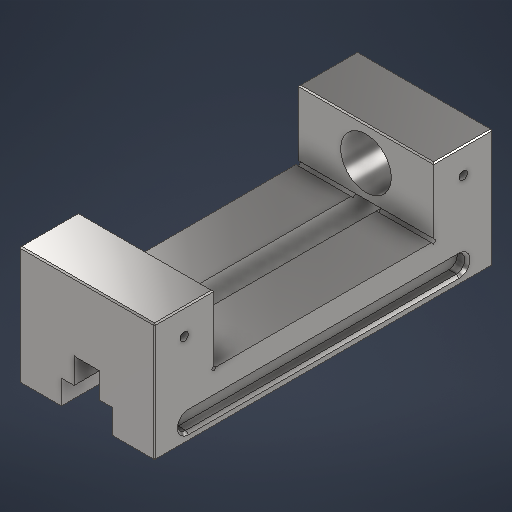
# Autodesk Inventor part: Part1
Saved by Autodesk Inventor 2026 (Build 300175000, 175)
## iProperties
Created: 2026-03-22
Part Number: Part1
Material: Generic
Document SubType Name: Modeling
Designer: Mlinč
Density: 1 g/cm^3
Appearance: Default
Author: Mlinč
Autodesk Inventor part; units mm, degrees
ref_plane "XZ Plane" through (0, 0, 0) normal (0, 1, 0) x (-1, 0, 0)
ref_plane "XY Plane" through (0, 0, 0) normal (0, 0, 1) x (1, 0, 0)
sketch "Sketch1" plane through (0, 0, 0) normal (0, 1, 0) x (-1, 0, 0)
  line L0 (0, 0) -> (80, 0)
  line L1 (80, 0) -> (80, -200)
  line L2 (80, -200) -> (0, -200)
  line L3 (0, -200) -> (0, 0)
  dimension "d0" = 80
  dimension "d1" = 200
  constraints: 8 end point, 2 parallel, 1 horizontal, 1 perpendicular
  measures "d0" distance of L0.start L0.end
  measures "d1" distance of L0.end L1.end
extrude "Extrusion1" add sketch "Sketch1" along normal blind 70
sketch "Sketch2" plane through (0, 0, 0) normal (1, 0, 0) x (0, 0, -1)
  line L0 (200, 70) -> (0, 70) projected
  line L1 (35, 70) -> (165, 70)
  line L2 (165, 70) -> (165, 30)
  line L3 (165, 30) -> (35, 30)
  line L4 (35, 30) -> (35, 70)
  line L5 (0, 0) -> (0, 70) projected
  line L6 (200, 0) -> (200, 70) projected
  dimension "d4" = 35
  dimension "d5" = 35
  dimension "d6" = 40
  constraints: 8 end point, 2 parallel, 1 horizontal, 1 perpendicular, 1 point on line
  measures "d4" distance between parallel lines of L5 L4
  measures "d5" distance between parallel lines of L6 L2
  measures "d6" distance of L3.end L1.start
extrude "Extrusion2" cut sketch "Sketch2" against normal through all
sketch "Sketch3" plane through (0, 0, -200) normal (0, 0, -1) x (-1, 0, 0)
  line L0 (80, 0) -> (0, 0) projected
  line L1 (25, 0) -> (25, 15)
  line L2 (25, 15) -> (32.5, 15)
  line L3 (32.5, 15) -> (32.5, 30)
  line L4 (32.5, 30) -> (47.5, 30)
  line L5 (47.5, 30) -> (47.5, 15)
  line L6 (47.5, 15) -> (55, 15)
  line L7 (55, 15) -> (55, 0)
  line L8 (40, 0) -> (40, 70) construction
  line L9 (80, 70) -> (0, 70) projected
  dimension "d9" = 15
  dimension "d10" = 15
  dimension "d11" = 30
  dimension "d12" = 15
  constraints: 16 end point, 5 perpendicular, 4 point on line, 2 midpoint, 1 collinear, 1 vertical, 1 other
  measures "d9" distance of L3.end L4.end
  measures "d10" distance of L1.start L1.end
  measures "d11" distance between parallel lines of L7 L1
  measures "d12" distance of L4.end L5.end
extrude "Extrusion3" cut sketch "Sketch3" against normal through all
sketch "Sketch4" plane through (0, 70, -200) normal (0, 0, -1) x (-1, 0, 0)
  circle A0 centre (40, -20) radius 15
  line L0 (0, 0) -> (80, 0) projected
  point P0 (0, -70)
  point P1 (40, 0)
  dimension "d15" = 20
  dimension "d16" = 30
  constraints: 1 centre point, 1 midpoint, 1 vertical alignment
  measures "d15" distance from line of L0 A0.centre
  measures "d16" diameter of A0
extrude "Extrusion4" cut sketch "Sketch4" against normal up to surface (35 mm away)
sketch "Sketch5" plane through (0, 0, 0) normal (1, 0, 0) x (0, 0, -1)
  line L0 (20, 10) -> (180, 10) construction
  line L1 (200, 15) -> (0, 15) projected
  line L2 (20, 5) -> (180, 5)
  line L3 (180, 15) -> (20, 15)
  arc A0 (20, 15) -> (20, 5) centre (20, 10) ccw
  arc A1 (180, 5) -> (180, 15) centre (180, 10) ccw
  line L4 (0, 0) -> (200, 0) projected
  line L5 (0, 0) -> (0, 70) projected
  point P0 (100, 10)
  dimension "d19" = 5
  dimension "d20" = 160
  dimension "d21" = 5
  dimension "d22" = 20
  constraints: 8 end point, 4 point on circle, 4 tangent, 2 centre point, 2 parallel, 1 midpoint
  measures "d19" radius of A0
  measures "d20" distance of L3.start L3.end
  measures "d21" distance between parallel lines of L2 L4
  measures "d22" distance from line of L5 L0.start
extrude "Extrusion5" cut sketch "Sketch5" against normal blind 6
ref_plane "Work Plane1" through (-40, 0, 0) normal (1, 0, 0) x (0, 1, 0)
mirror "Mirror1" about plane through (-40, 0, 0) normal (1, 0, 0) of "Extrusion5"
sketch "Sketch6" plane through (0, 0, 0) normal (1, 0, 0) x (0, 0, -1)
  line L0 (35, 28.5858) -> (33.5858, 30)
  line L1 (33.5858, 30) -> (35, 31.4142)
  line L2 (35, 31.4142) -> (36.4142, 30)
  line L3 (36.4142, 30) -> (35, 28.5858)
  line L4 (165, 30) -> (35, 30) projected
  line L5 (35, 28.5858) -> (35, 31.4142) construction
  line L6 (33.5858, 30) -> (36.4142, 30) construction
  line L7 (165, 28.5858) -> (166.4142, 30)
  line L8 (166.4142, 30) -> (165, 31.4142)
  line L9 (165, 31.4142) -> (163.5858, 30)
  line L10 (163.5858, 30) -> (165, 28.5858)
  line L11 (165, 28.5858) -> (165, 31.4142) construction
  line L12 (166.4142, 30) -> (163.5858, 30) construction
  point P0 (0, 0)
  dimension "d26" = 2
  constraints: 24 end point, 5 perpendicular, 4 midpoint, 4 parallel, 2 horizontal
  measures "d26" distance of L1.end L2.end
extrude "Extrusion6" cut sketch "Sketch6" against normal through all
sketch "Sketch7" plane through (0, 0, 0) normal (1, 0, 0) x (0, 0, -1)
  circle A0 centre (17.5, 55) radius 2.5
  circle A1 centre (182.5, 55) radius 2.5
  line L0 (0, 70) -> (35, 70) projected
  line L1 (0, 0) -> (0, 70) projected
  line L2 (200, 0) -> (200, 70) projected
  dimension "d30" = 5
  dimension "d31" = 15
  dimension "d32" = 17.5
  dimension "d33" = 17.5
  constraints: 2 centre point, 1 equal radius, 1 horizontal alignment
  measures "d30" diameter of A0
  measures "d31" distance from line of L0 A0.centre
  measures "d32" distance from line of L1 A0.centre
  measures "d33" distance from line of L2 A1.centre
extrude "Extrusion7" cut sketch "Sketch7" against normal blind 18
mirror "Mirror2" about plane through (-40, 0, 0) normal (1, 0, 0) of "Extrusion7"
chamfer "Chamfer1" distance 1.5 angle 45 8 edges at (-80, 5, -100) (-80, 10, -185) (-80, 15, -100) (-80, 10, -15) (0, 5, -100) (0, 10, -15) (0, 15, -100) (0, 10, -185)
chamfer "Chamfer2" distance 0.75 angle 45 20 edges at (-40, 70, -165) (0, 70, -182.5) (-40, 70, -200) (-80, 70, -182.5) (-80, 35, -200) (0, 35, -200) (-67.5, 0, -200) (-12.5, 0, -200) (-25, 0, -100) (-55, 0, -100) (-80, 0, -100) (0, 0, -100) (-12.5, 0, 0) (-67.5, 0, 0) (-80, 35, 0) (0, 35, 0) (-40, 70, 0) (0, 70, -17.5) (-40, 70, -35) (-80, 70, -17.5)
thread "Thread1" size "M6x1" class "6H" standard "ANSI Metric M Profile" length 15 offset 3
thread "Thread2" size "M5x0.8" class "6H" standard "ANSI Metric M Profile" length 15
thread "Thread3" size "M5x0.8" class "6H" standard "ANSI Metric M Profile" length 15
thread "Thread4" size "M5x0.8" class "6H" standard "ANSI Metric M Profile" length 15
sketch "Sketch9" plane through (-47.5, 30, -200) normal (0, -1, 0) x (1, 0, 0)
  circle A0 centre (7.5, 15) radius 2.5
  line L0 (15, 0) -> (0, 0) projected
  line L1 (0, 0) -> (0, 200) projected
  point P0 (47.5, 200)
  dimension "d55" = 15
  dimension "d56" = 5
  dimension "d57" = 7.5
  constraints: 1 centre point
  measures "d55" distance from line of L0 A0.centre
  measures "d56" diameter of A0
  measures "d57" distance from line of L1 A0.centre
extrude "Extrusion8" cut sketch "Sketch9" against normal up to surface
thread "Thread5" size "M6x1" class "6H" standard "ANSI Metric M Profile" full length
body "Solid1"
